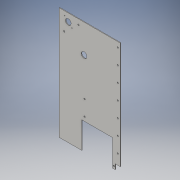
# Autodesk Inventor part: GearboxPlateRev2
Saved by Autodesk Inventor 2016 (Build 200138000, 138)
## iProperties
Created: 2017-01-22
Part Number: GearboxPlateRev2
Material: Generic
Document SubType Name: Modeling
Designer: madsenn
Density: 1 g/cm^3
Appearance: Default
Author: madsenn
Autodesk Inventor part; units mm, degrees
ref_plane "YZ Plane" through (0, 0, 0) normal (1, 0, 0) x (0, 1, 0)
ref_plane "XZ Plane" through (0, 0, 0) normal (0, 1, 0) x (-1, 0, 0)
ref_plane "XY Plane" through (0, 0, 0) normal (0, 0, 1) x (1, 0, 0)
sketch "Sketch1" plane through (0, 0, 0) normal (0, 0, 1) x (1, 0, 0)
  line L0 (-115.6368, 165.4342) -> (189.1632, 165.4342)
  line L1 (189.1632, 165.4342) -> (189.1632, -393.3658)
  line L2 (189.1632, -393.3658) -> (-115.6368, -393.3658)
  line L3 (-115.6368, -393.3658) -> (-115.6368, 165.4342)
  line L4 (151.0632, -393.3658) -> (151.0632, -261.2858)
  line L5 (189.1632, -393.3658) -> (163.5092, -393.3658)
  line L6 (163.5092, -393.3658) -> (163.5092, -367.7118)
  line L7 (163.5092, -367.7118) -> (189.1632, -367.7118)
  line L8 (189.1632, -367.7118) -> (189.1632, -393.3658)
  line L9 (151.0632, -261.2858) -> (-3.064, -261.2858)
  line L10 (-3.064, -261.2858) -> (-3.064, -393.3658)
  circle A0 centre (157.2862, -380.5388) radius 3.5687
  line L11 (189.1632, -317.1658) -> (-115.6368, -317.1658)
  circle A1 centre (9.0264, 24.007) radius 14.2875
  point P0 (0, 0)
  dimension "d0" = 304.8
  dimension "d1" = 558.8
  dimension "d2" = 180.1368
  dimension "d3" = 417.3728
  dimension "d4" = 38.1
  dimension "d5" = 25.654
  dimension "d6" = 25.654
  dimension "d7" = 154.1272
  dimension "d10" = 132.08
  dimension "d11" = 12.446
  dimension "d12" = 6.223
  dimension "d13" = 12.827
  dimension "d14" = 7.1374
  dimension "d15" = 76.2
  dimension "d16" = 28.575
  constraints: 24 end point, 4 parallel, 4 perpendicular, 4 point on line, 3 horizontal, 2 centre point, 2 coincident, 1 vertical
  measures "d0" distance of L0.start L0.end
  measures "d1" distance of L2.end L0.start
  measures "d2" distance from line of point (9.026, 24.007) L1
  measures "d3" distance from line of L2 point (9.026, 24.007)
  measures "d4" distance between parallel lines of L1 L4
  measures "d5" distance of L6.end L7.end
  measures "d6" distance between parallel lines of L2 L7
  measures "d7" distance of L4.end L9.end
  measures "d10" distance of L9.end L10.end
  measures "d11" distance between parallel lines of L6 L4
  measures "d12" distance from line of L6 point (157.286, -380.539)
  measures "d13" distance from line of L2 point (157.286, -380.539)
  measures "d14" diameter of A0
  measures "d15" distance between parallel lines of L2 L11
  measures "d16" diameter of A1
extrude "Extrusion1" add sketch "Sketch1" along normal blind 3.175 contours L0 L1 L11 L4 L9 L10 L3 | L11 L10 L2 L3 | L1 L7 L6 L2 L4 L11
sketch "Sketch2" plane through (0, 0, 3.175) normal (0, 0, 1) x (1, 0, 0)
  line L0 (151.0632, -393.3658) -> (163.5092, -393.3658) projected
  line L1 (189.1632, -367.7118) -> (189.1632, 165.4342) projected
  point P0 (0, 0)
  point P1 (176.4632, -317.1658)
  point P2 (176.4632, -240.9658)
  point P3 (176.4632, -164.7658)
  point P4 (176.4632, -88.5658)
  point P5 (176.4632, -12.3658)
  point P6 (176.4632, 63.8342)
  point P7 (176.4632, 140.0342)
  point P8 (11.3632, -240.9658)
  point P9 (11.3632, -164.7658)
  dimension "d20" = 76.2
  dimension "d21" = 12.7
  dimension "d22" = 76.2
  dimension "d23" = 76.2
  dimension "d24" = 76.2
  dimension "d25" = 76.2
  dimension "d26" = 76.2
  dimension "d27" = 76.2
  dimension "d29" = 165.1
  dimension "d30" = 165.1
  measures "d20" distance from line of L0 point (176.463, -317.166)
  measures "d21" distance from line of point (176.463, -317.166) L1
  measures "d22" distance of point (176.463, -240.966) point (176.463, -317.166)
  measures "d23" distance of point (176.463, -240.966) point (176.463, -164.766)
  measures "d24" distance of point (176.463, -164.766) point (176.463, -88.566)
  measures "d25" distance of point (176.463, -88.566) point (176.463, -12.366)
  measures "d26" distance of point (176.463, -12.366) point (176.463, 63.834)
  measures "d27" distance of point (176.463, 63.834) point (176.463, 140.034)
  measures "d29" distance of point (176.463, -240.966) point (11.363, -240.966)
  measures "d30" distance of point (176.463, -164.766) point (11.363, -164.766)
hole "Hole1" at (176.4632, -317.1658, 3.175) at (176.4632, -240.9658, 3.175) at (176.4632, -164.7658, 3.175) at (176.4632, -88.5658, 3.175) at (176.4632, -12.3658, 3.175) at (176.4632, 63.8342, 3.175) at (176.4632, 140.0342, 3.175) at (11.3632, -240.9658, 3.175) at (11.3632, -164.7658, 3.175) direction (0, 0, -1) diameter 7.1374 end through all
sketch "Sketch4" plane through (0, 0, 3.175) normal (0, 0, 1) x (1, 0, 0)
  circle A0 centre (-69.9042, 127.3342) radius 14.195
  circle A1 centre (-87.8647, 145.2947) radius 2.0193
  circle A2 centre (-51.9436, 109.3737) radius 2.0193
  line L0 (-90.9042, 134.5342) -> (-90.9042, 120.1342)
  line L1 (-90.9042, 120.1342) -> (-92.1292, 118.9092)
  line L2 (-92.1292, 118.9092) -> (-92.1292, 113.3342)
  line L3 (-92.1292, 113.3342) -> (-85.9042, 113.3342)
  arc A3 (-83.9042, 111.3342) -> (-85.9042, 113.3342) centre (-85.9042, 111.3342) ccw
  line L4 (-83.9042, 111.3342) -> (-83.9042, 106.3342)
  line L5 (-83.9042, 106.3342) -> (-49.9042, 106.3342)
  arc A4 (-49.9042, 106.3342) -> (-48.9042, 107.3342) centre (-69.9042, 127.3342) ccw
  line L6 (-48.9042, 107.3342) -> (-48.9042, 109.1342)
  line L7 (-48.9042, 109.1342) -> (-47.6792, 110.3592)
  line L8 (-47.6792, 110.3592) -> (-47.6792, 118.9092)
  line L9 (-47.6792, 118.9092) -> (-48.9042, 120.1342)
  line L10 (-48.9042, 120.1342) -> (-48.9042, 134.5342)
  line L11 (-48.9042, 134.5342) -> (-47.6792, 135.7592)
  line L12 (-47.6792, 135.7592) -> (-47.6792, 141.3342)
  line L13 (-47.6792, 141.3342) -> (-53.9042, 141.3342)
  arc A5 (-55.9042, 143.3342) -> (-53.9042, 141.3342) centre (-53.9042, 143.3342) ccw
  line L14 (-55.9042, 143.3342) -> (-55.9042, 148.3342)
  line L15 (-55.9042, 148.3342) -> (-89.9042, 148.3342)
  arc A6 (-89.9042, 148.3342) -> (-90.9042, 147.3342) centre (-69.9042, 127.3342) ccw
  line L16 (-90.9042, 147.3342) -> (-90.9042, 145.5342)
  line L17 (-90.9042, 145.5342) -> (-92.1292, 144.3092)
  line L18 (-92.1292, 144.3092) -> (-92.1292, 135.7592)
  line L19 (-92.1292, 135.7592) -> (-90.9042, 134.5342)
  circle A7 centre (9.0264, 24.007) radius 14.2875 projected
  line L20 (189.1632, 165.4342) -> (-115.6368, 165.4342) projected
  line L21 (-115.6368, 165.4342) -> (-115.6368, -393.3658) projected
  point P0 (0, 0)
  dimension "d50" = 3.0395
  dimension "d51" = 4.2645
  dimension "d52" = 4.2645
  dimension "d53" = 3.0395
  dimension "d54" = 130.0251
  dimension "d55" = 21
  dimension "d56" = 21
  dimension "d57" = 38.1
  dimension "d59" = 45.7327
  constraints: 40 end point, 8 point on circle, 7 centre point
  measures "d50" distance from line of L15 A1.centre
  measures "d51" distance from line of L18 A1.centre
  measures "d52" distance from line of L8 A2.centre
  measures "d53" distance from line of L5 A2.centre
  measures "d54" distance of A7.centre A0.centre
  measures "d55" distance from line of L5 A0.centre
  measures "d56" distance from line of L0 A0.centre
  measures "d57" distance from line of L20 A0.centre
  measures "d59" distance from line of L21 A0.centre
extrude "Extrusion3" cut sketch "Sketch4" against normal blind 25.4 contours A0 | A1 | A2
sketch "Sketch5" plane through (0, 0, 3.175) normal (0, 0, 1) x (1, 0, 0)
  line L0 (-115.6368, 165.4342) -> (-115.6368, -393.3658) projected
  line L1 (189.1632, 165.4342) -> (-115.6368, 165.4342) projected
  circle A0 centre (-69.9042, 127.3342) radius 14.195 projected
  point P0 (0, 0)
  point P1 (-90.2368, 76.5342)
  point P2 (-19.1042, 140.0342)
  dimension "d62" = 25.4
  dimension "d63" = 25.4
  dimension "d64" = 50.8
  dimension "d65" = 50.8
  measures "d62" distance from line of L0 point (-90.237, 76.534)
  measures "d63" distance from line of L1 point (-19.104, 140.034)
  measures "d64" horizontal distance of A0.centre point (-19.104, 140.034)
  measures "d65" vertical distance of point (-90.237, 76.534) A0.centre
hole "Hole2" at (-90.2368, 76.5342, 3.175) at (-19.1042, 140.0342, 3.175) direction (0, 0, -1) diameter 7.1374 end through all
body "Solid1"
